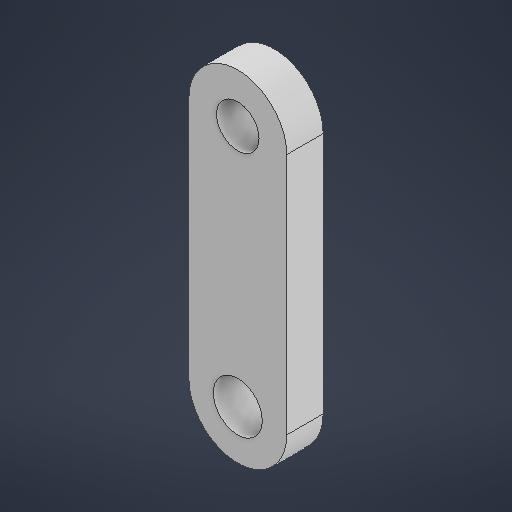
# Autodesk Inventor part: RedKangoroo_001_bar1ipt
Saved by Autodesk Inventor 2026.3 (Build 303398000, 398)
## iProperties
Created: 2026-05-22
Part Number: RedKangoroo_001_bar1ipt
Material: Generic
Document SubType Name: Modeling
Designer: ADMIN
Density: 1 g/cm^3
Appearance: Default
Author: ADMIN
Autodesk Inventor part; units mm, degrees
ref_plane "YZ Plane" through (0, 0, 0) normal (1, 0, 0) x (0, 1, 0)
ref_plane "XZ Plane" through (0, 0, 0) normal (0, 1, 0) x (-1, 0, 0)
ref_plane "XY Plane" through (0, 0, 0) normal (0, 0, 1) x (1, 0, 0)
sketch "Sketch1" plane through (0, 0, 0) normal (0, 0, 1) x (1, 0, 0)
  line L0 (0, 0) -> (0, 20) construction
  circle A0 centre (0, 0) radius 2.02
  circle A1 centre (0, 20) radius 1.75
  line L1 (0, 0) -> (0, 20) construction
  line L2 (4.0329, 0) -> (4.0329, 20)
  line L3 (-4.0329, 20) -> (-4.0329, 0)
  arc A2 (-4.0329, 0) -> (4.0329, 0) centre (0, 0) ccw
  arc A3 (4.0329, 20) -> (-4.0329, 20) centre (0, 20) ccw
  point P0 (0, 10)
  point P1 (0, 10)
  dimension "d0" = 20
  dimension "d2" = 4.04
  dimension "d3" = 3.5
  constraints: 12 end point, 4 centre point, 4 point on circle, 4 tangent, 2 coincident, 2 equal length, 2 midpoint, 1 vertical
  measures "d0" distance of L0.start L0.end
  measures "d2" diameter of A0
  measures "d3" diameter of A1
extrude "Extrusion2" add sketch "Sketch1" along normal blind 3
body "Solid2"
